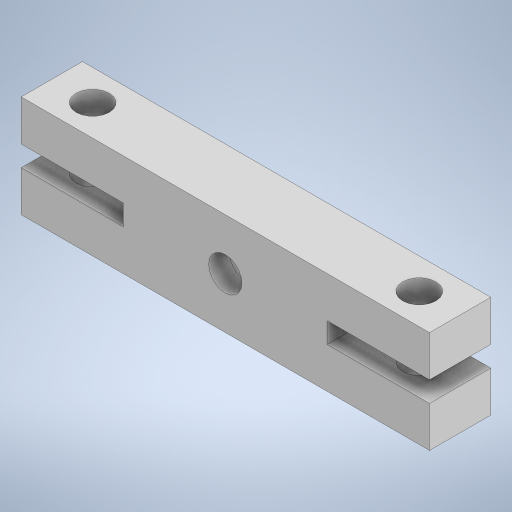
# Autodesk Inventor part: Connector
Saved by Autodesk Inventor 2023 (Build 270158000, 158)
## iProperties
Created: 2023-02-27
Part Number: Connector
Material: Generic
Document SubType Name: Modeling
Designer: Gabriel - T3 CAD
Density: 1 g/cm^3
Appearance: Default
Author: Gabriel - T3 CAD
Autodesk Inventor part; units mm, degrees
ref_plane "YZ Plane" through (0, 0, 0) normal (1, 0, 0) x (0, 1, 0)
ref_plane "XZ Plane" through (0, 0, 0) normal (0, 1, 0) x (-1, 0, 0)
ref_plane "XY Plane" through (0, 0, 0) normal (0, 0, 1) x (1, 0, 0)
sketch "Sketch1" plane through (0, 0, 0) normal (0, 0, 1) x (1, 0, 0)
  line L0 (0, 0) -> (-63.5, 0)
  line L1 (-63.5, 0) -> (-63.5, 15.875)
  line L2 (-63.5, 15.875) -> (0, 15.875)
  line L3 (0, 15.875) -> (0, 0)
  line L4 (0, 6.35) -> (-63.5, 6.35)
  line L5 (-63.5, 6.35) -> (-63.5, 9.525)
  line L6 (-63.5, 9.525) -> (0, 9.525)
  line L7 (0, 9.525) -> (0, 6.35)
  line L8 (-47.625, 15.875) -> (-15.875, 15.875)
  line L9 (-15.875, 15.875) -> (-15.875, 0)
  line L10 (-15.875, 0) -> (-47.625, 0)
  line L11 (-47.625, 0) -> (-47.625, 15.875)
  circle A0 centre (-31.75, 7.9375) radius 6.35
  circle A1 centre (-31.75, 7.9375) radius 2.5797
  line L12 (-6.35, 6.35) -> (-6.35, 9.525)
  line L13 (-57.15, 6.35) -> (-57.15, 9.525)
  point P0 (-15.875, 6.35)
  point P1 (-15.875, 9.525)
  point P2 (-47.625, 9.525)
  point P3 (-47.625, 6.35)
  dimension "d12" = 15.875
  dimension "d13" = 6.35
  dimension "d14" = 3.175
  dimension "d15" = 15.875
  dimension "d16" = 15.875
  dimension "d17" = 7.9375
  dimension "d18" = 31.75
  dimension "d19" = 12.7
  dimension "d20" = 5.1594
  dimension "d33" = 6.35
  dimension "d34" = 6.35
  dimension "d35" = 50.8
  dimension "d36" = 63.5
  constraints: 28 end point, 8 point on line, 6 parallel, 4 perpendicular, 3 horizontal, 2 centre point, 1 coincident, 1 vertical
  measures "d12" distance of L0.end L1.end
  measures "d13" distance between parallel lines of L0 L4
  measures "d14" distance between parallel lines of L6 L4
  measures "d15" distance between parallel lines of L1 L11
  measures "d16" distance between parallel lines of L3 L9
  measures "d17" distance from line of L10 A0.centre
  measures "d18" distance from line of L1 A0.centre
  measures "d19" diameter of A0
  measures "d20" diameter of A1
  measures "d33" distance between parallel lines of L7 L12
  measures "d34" distance between parallel lines of L5 L13
  measures "d35" distance between parallel lines of L13 L12
  measures "d36" distance between parallel lines of L1 L3
extrude "Extrusion1" add sketch "Sketch1" along normal blind 9.525 contours L0 L9 L4 L3 | L0 L11 L4 A0 L9 | L0 L1 L4 L11 | L4 A0 L6 L9 | L6 L9 L2 L3 | L11 L6 A0 L4 | A0 L4 A1 | L4 A1 L6 A0 | L6 A0 L11 L2 L9 | A0 L6 A1 L4 | L6 L1 L2 L11 | L6 A1 A0
extrude "Extrusion2" cut sketch "Sketch1" along normal blind 6.35 contours A0 L4 A1 | L4 A1 L6 A0 | A0 L6 A1 L4 | A1 L4 | L4 A1 L6 | L6 A1 A0 | L6 A1
sketch "Sketch2" plane through (-63.5, 15.875, 0) normal (0, 1, 0) x (1, 0, 0)
  circle A0 centre (57.15, -4.7625) radius 2.5797
  circle A1 centre (6.35, -4.7625) radius 2.5797
  line L0 (63.5, 0) -> (0, 0) projected
  line L1 (63.5, 0) -> (63.5, -9.525) projected
  line L2 (0, 0) -> (0, -9.525) projected
  dimension "d25" = 4.7625
  dimension "d26" = 4.7625
  dimension "d27" = 6.35
  dimension "d28" = 6.35
  dimension "d29" = 5.1594
  constraints: 2 centre point, 1 equal radius
  measures "d25" distance from line of L0 A0.centre
  measures "d26" distance from line of L0 A1.centre
  measures "d27" distance from line of L1 A0.centre
  measures "d28" distance from line of L2 A1.centre
  measures "d29" diameter of A0
extrude "Extrusion3" cut sketch "Sketch2" against normal through all
equation "\"d16\" = d15"
equation "\"d17\" = 0.5 * d12"
equation "\"d18\" = 0.5 * d36"
equation "\"d33\" = d34"
equation "\"d34\" = d13"
equation "\"d26\" = d25"
equation "\"d27\" = d28"
body "Solid1"
